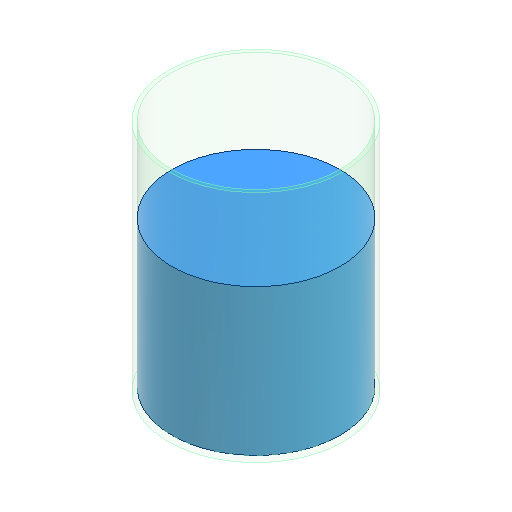
# Autodesk Inventor part: water-tank-sizing-by-calcslive-plug
Saved by Autodesk Inventor 2026.1 (Build 301233020, 233B)
## iProperties
Created: 2026-01-01
Part Number: water-tank-sizing-by-calcslive-plug
Material: Generic
Document SubType Name: Modeling
Designer: holy
Density: 1 g/cm^3
Appearance: Default
Author: holy
Autodesk Inventor part; units mm, degrees
ref_plane "YZ Plane" through (0, 0, 0) normal (1, 0, 0) x (0, 1, 0)
ref_plane "XZ Plane" through (0, 0, 0) normal (0, 1, 0) x (-1, 0, 0)
ref_plane "XY Plane" through (0, 0, 0) normal (0, 0, 1) x (1, 0, 0)
sketch "Sketch1" plane through (0, 0, 0) normal (0, 0, 1) x (1, 0, 0)
  line L0 (-30.48, 0) -> (182.88, 0) construction
  line L1 (0, -81.28) -> (0, 487.68) construction
  line L2 (146.05, 406.4) -> (152.4, 406.4)
  line L3 (152.4, 406.4) -> (152.4, 6.35)
  line L4 (152.4, 6.35) -> (146.05, 6.35)
  line L5 (146.05, 6.35) -> (146.05, 406.4)
  line L6 (0, 0) -> (152.4, 0)
  line L7 (152.4, 0) -> (152.4, 6.35)
  line L8 (152.4, 6.35) -> (0, 6.35)
  line L9 (0, 6.35) -> (0, 0)
  line L10 (0, 260.35) -> (146.05, 260.35)
  line L11 (146.05, 260.35) -> (146.05, 6.35)
  line L12 (146.05, 6.35) -> (0, 6.35)
  line L13 (0, 6.35) -> (0, 260.35)
  point P0 (146.05, 6.35)
  point P1 (0, 6.35)
  point P2 (146.05, 260.35)
  dimension "d0" = 152.4
  dimension "d1" = 406.4
  dimension "d2" = 6.35
  dimension "d3" = 254
  constraints: 24 end point, 6 parallel, 5 collinear, 4 perpendicular, 3 horizontal
  measures "d0" distance of L6.start L6.end
  measures "d1" distance between parallel lines of L2 L6
  measures "d2" distance of L2.start L2.end
  measures "d3" distance of L12.end L10.start
revolve "Revolution1" add sketch "Sketch1" angle 360 about axis through (0, 6.35, 0) along (0, 1, 0) contours L2 L3 L4 L5 | L7 L6 L9 L8 L4
revolve "Revolution2" add sketch "Sketch1" angle 360 about axis through (0, -10, 0) along (0, 1, 0) separate body contours L5 L8 L13 L10
equation "\"d0\" = 0.5 * BaseDia"
equation "\"d1\" = Height"
equation "\"d2\" = Thickness"
equation "\"d3\" = LiquidDepth"
equation "\"BaseDia\" = 304.8"
equation "\"Height\" = 406.4"
equation "\"Thickness\" = 6.35"
equation "\"LiquidDepth\" = 254"
